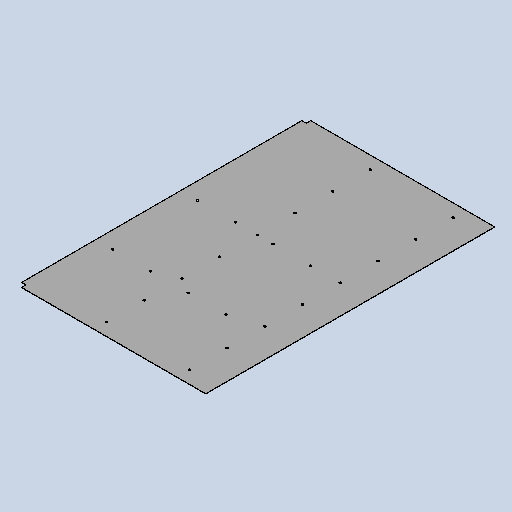
# Autodesk Inventor part: GnG R.1 floor sheet
Saved by Autodesk Inventor 2025.3 (Build 293356030, 356C)
## iProperties
Created: 2025-10-28
Part Number: GnG R.1 floor sheet
Material: Stainless Steel
Document SubType Name: Sheet Metal
Designer: admin
Stock Number: R 1
Mass: 82638.7 g
Surface Area: 69127.8 cm^2
Volume: 10329.8 cm^3
Density: 8 g/cm^3
Flat Pattern Width: 150 cm
Flat Pattern Length: 230 cm
Flat Pattern Area: 34500 cm^2
Sheet Metal Rule: AISI304 3mm Die 32
Sheet Metal Width: 1500,000 mm
Sheet Metal Length: 2300,000 mm
Sheet Metal Area: 3450000,000 mm^2
Appearance: Default
Author: admin
Autodesk Inventor part; units mm, degrees
ref_plane "YZ Plane" through (0, 0, 0) normal (1, 0, 0) x (0, 1, 0)
ref_plane "XZ Plane" through (0, 0, 0) normal (0, 1, 0) x (-1, 0, 0)
ref_plane "XY Plane" through (0, 0, 0) normal (0, 0, 1) x (1, 0, 0)
sketch "Sketch1" plane through (0, 0, 0) normal (0, 0, 1) x (1, 0, 0)
  line L0 (0, 0) -> (-1500, 0)
  line L1 (-1500, 0) -> (-1500, -2300)
  line L2 (-1500, -2300) -> (0, -2300)
  line L3 (0, -2300) -> (0, 0)
  line L4 (0, 0) -> (-35, 0)
  line L5 (-35, 0) -> (-35, -35)
  line L6 (-35, -35) -> (0, -35)
  line L7 (0, -35) -> (0, 0)
  line L8 (0, -2300) -> (-35, -2300)
  line L9 (-35, -2300) -> (-35, -2265)
  line L10 (-35, -2265) -> (0, -2265)
  line L11 (0, -2265) -> (0, -2300)
  line L12 (-1500, 0) -> (-1465, 0)
  line L13 (-1465, 0) -> (-1465, -35)
  line L14 (-1465, -35) -> (-1500, -35)
  line L15 (-1500, -35) -> (-1500, 0)
  line L16 (-1500, -2300) -> (-1465, -2300)
  line L17 (-1465, -2300) -> (-1465, -2265)
  line L18 (-1465, -2265) -> (-1500, -2265)
  line L19 (-1500, -2265) -> (-1500, -2300)
  line L20 (-1435, -2300) -> (-1345, -2300)
  line L21 (-1345, -2300) -> (-1345, -2265)
  line L22 (-1345, -2265) -> (-1435, -2265)
  line L23 (-1435, -2265) -> (-1435, -2300)
  line L24 (-1435, 0) -> (-1345, 0)
  line L25 (-1345, 0) -> (-1345, -35)
  line L26 (-1345, -35) -> (-1435, -35)
  line L27 (-1435, -35) -> (-1435, 0)
  point P0 (0, -35)
  point P1 (0, -2265)
  point P2 (-1345, 0)
  point P3 (-1465, 0)
  point P4 (-1500, -35)
  dimension "d22" = 1500
  dimension "d23" = 2300
  dimension "d24" = 35
  dimension "d25" = 35
  dimension "d28" = 90
  dimension "d29" = 1310
  measures "d22" distance of L2.end L1.end
  measures "d23" distance of L1.end L0.end
  measures "d24" distance of L6.end L5.end
  measures "d25" distance of L5.end L4.end
  measures "d28" distance of L25.end L26.end
  measures "d29" distance between parallel lines of L5 L25
extrude "Plate1" add sketch "Sketch1" along normal blind 3 contours L3 L6 L5 L0 | L5 L6 L3 L10 L9 L2 L21 L22 L23 L17 L18 L1 L14 L13 L0 L27 L26 L25 | L25 L26 L27 L0 | L3 L2 L9 L10 | L2 L23 L22 L21
sketch "Sketch5" plane through (0, 0, 3) normal (0, 0, 1) x (1, 0, 0)
  circle A0 centre (-77.6102, 0) radius 2.5
  line L0 (-130.4089, -2) -> (-130.4089, 0)
  line L1 (-130.4089, 0) -> (-125.4089, 0)
  line L2 (-125.4089, 0) -> (-125.4089, -2)
  line L3 (-125.4089, -2) -> (-130.4089, -2)
  line L4 (-125.4089, -1) -> (-120.4089, -1) construction
  line L5 (-120.4089, -2) -> (-120.4089, 0)
  line L6 (-115.4089, -2) -> (-120.4089, -2)
  line L7 (-120.4089, 0) -> (-115.4089, 0)
  line L8 (-115.4089, 0) -> (-115.4089, -2)
  line L9 (-115.4089, -1) -> (-110.4089, -1) construction
  line L10 (-110.4089, -2) -> (-110.4089, 0)
  line L11 (-110.4089, 0) -> (-105.4089, 0)
  line L12 (-105.4089, 0) -> (-105.4089, -2)
  line L13 (-105.4089, -2) -> (-110.4089, -2)
  line L14 (-1465, 0) -> (0, 0) projected
  line L15 (-95.4089, -2) -> (-100.4089, -2)
  line L16 (-100.4089, -2) -> (-100.4089, 0)
  line L17 (-95.4089, 0) -> (-95.4089, -2)
  line L18 (-100.4089, 0) -> (-95.4089, 0)
  line L19 (-100.4089, -1) -> (-105.4089, -1)
  circle A1 centre (-66.0411, 0) radius 2.5
  point P0 (-97.9089, 0)
  point P1 (-95.4089, 0)
  point P2 (-100.4089, 0)
  point P3 (-63.5411, 0)
  point P4 (-68.5411, 0)
  dimension "d34" = 5
  dimension "d35" = 2
  dimension "d36" = 5
  dimension "d41" = 5
  constraints: 38 end point, 8 parallel, 7 horizontal, 7 midpoint, 6 equal length, 4 perpendicular, 3 collinear, 3 point on line, 2 centre point
  measures "d34" distance of L2.end L0.start
  measures "d35" distance of L0.start L0.end
  measures "d36" diameter of A0
  measures "d41" diameter of A1
extrude "Cut1" cut sketch "Sketch5" against normal blind 3 contours L14 A0 | L17 L15 L16 L14 | A0 L14 | L14 A1 picked at (-66.3006, -1.5131)
sketch "Sketch6" plane through (0, 0, 3) normal (0, 0, 1) x (1, 0, 0)
  line L0 (0, -2300) -> (0, 0) construction
  line L1 (-1465, -2300) -> (0, -2300) construction
  line L2 (-230, -2300) -> (-230, -100) construction
  line L3 (-890, -2300) -> (-890, -100) construction
  line L4 (0, -1000) -> (-1365, -1000) construction
  line L5 (-230, -1675) -> (-1365, -1675) construction
  circle A0 centre (-230, -100) radius 7.5
  circle A1 centre (-890, -100) radius 7.5
  circle A2 centre (-230, -400) radius 7.5
  circle A3 centre (-890, -400) radius 7.5
  circle A4 centre (-230, -700) radius 7.5
  circle A5 centre (-890, -700) radius 7.5
  circle A6 centre (-230, -1000) radius 7.5
  circle A7 centre (-890, -1000) radius 7.5
  circle A8 centre (-230, -1300) radius 7.5
  circle A9 centre (-890, -1300) radius 7.5
  circle A10 centre (-230, -1600) radius 7.5
  circle A11 centre (-890, -1600) radius 7.5
  circle A12 centre (-230, -1900) radius 7.5
  circle A13 centre (-890, -1900) radius 7.5
  circle A14 centre (-230, -2200) radius 7.5
  circle A15 centre (-890, -2200) radius 7.5
  circle A16 centre (-230, -2500) radius 7.5
  circle A17 centre (-890, -2500) radius 7.5
  circle A18 centre (-230, -2800) radius 7.5
  circle A19 centre (-890, -2800) radius 7.5
  circle A20 centre (-230, -3100) radius 7.5
  circle A21 centre (-890, -3100) radius 7.5
  circle A22 centre (-1365, -1675) radius 7.5
  circle A23 centre (-1365, -1000) radius 7.5
  circle A24 centre (-1065, -1675) radius 7.5
  circle A25 centre (-1065, -1000) radius 7.5
  circle A26 centre (-765, -1675) radius 7.5
  circle A27 centre (-765, -1000) radius 7.5
  circle A28 centre (-465, -1675) radius 7.5
  circle A29 centre (-465, -1000) radius 7.5
  dimension "d42" = 230
  dimension "d43" = 625
  dimension "d44" = 660
  dimension "d45" = 675
  dimension "d46" = 15
  dimension "d49" = 300
  dimension "d54" = 100
  dimension "d55" = -800
  dimension "d56" = 100
  dimension "d59" = 300
  constraints: 30 centre point, 30 coincident, 8 end point, 4 perpendicular, 4 point on line, 3 equal radius, 1 horizontal, 1 horizontal alignment, 1 vertical, 1 vertical alignment, 78 other
  measures "d42" distance between parallel lines of L0 L2
  measures "d43" distance between parallel lines of L1 L5
  measures "d44" distance between parallel lines of L2 L3
  measures "d45" distance between parallel lines of L5 L4
  measures "d46" diameter of A0
  measures "d49" distance of L2.end point (-230, -400)
  measures "d54" vertical distance of L2.end L0.end
  measures "d55" distance from line of L1 point (-230, -3100)
  measures "d56" horizontal distance of L5.end L1.start
  measures "d59" distance of L4.end point (-1065, -1000)
extrude "Cut2" cut sketch "Sketch6" against normal blind 3
equation "\"d24\" = d25"
equation "\"d39\" = Thickness"
equation "\"d56\" = d54"
equation "\"d64\" = Thickness"
equation "\"d2\" = Thickness"
equation "\"BendReliefWidth\" = Thickness"
equation "\"BendReliefDepth\" = 0.5 * Thickness"
equation "\"CornerReliefSize\" = 4 * Thickness"
equation "\"MinimumRemnant\" = 2 * Thickness"
equation "\"TransitionRadius\" = BendRadius"
equation "\"JacobiRadiusSize\" = BendRadius"
equation "\"GapSize\" = Thickness"
equation "\"Thickness\" = 3"
equation "\"BendRadius\" = 5"
body "Solid1"
